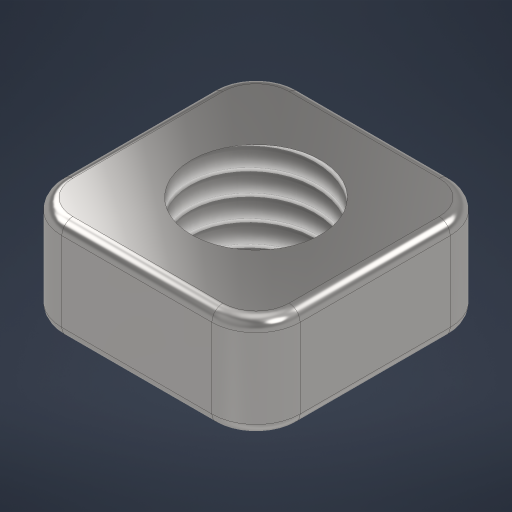
# Autodesk Inventor part: M3 Square Nut
Saved by Autodesk Inventor 2024 (Build 280153000, 153)
## iProperties
Created: 2024-10-26
Part Number: M3 Square Nut
Material: Generic
Document SubType Name: Modeling
Designer: jerem
Density: 1 g/cm^3
Appearance: Default
Author: jerem
Autodesk Inventor part; units mm, degrees
ref_plane "YZ Plane" through (0, 0, 0) normal (1, 0, 0) x (0, 1, 0)
ref_plane "XZ Plane" through (0, 0, 0) normal (0, 1, 0) x (-1, 0, 0)
ref_plane "XY Plane" through (0, 0, 0) normal (0, 0, 1) x (1, 0, 0)
sketch "Sketch1" plane through (0, 0, 0) normal (0, 1, 0) x (-1, 0, 0)
  circle A0 centre (0, 0) radius 1.465
  line L0 (-1.7, -2.7) -> (1.7, -2.7)
  line L1 (2.7, -1.7) -> (2.7, 1.7)
  line L2 (1.7, 2.7) -> (-1.7, 2.7)
  line L3 (-2.7, 1.7) -> (-2.7, -1.7)
  line L4 (-2.7, -2.7) -> (2.7, 2.7) construction
  line L5 (2.7, -2.7) -> (-2.7, 2.7) construction
  arc A1 (2.7, 1.7) -> (1.7, 2.7) centre (1.7, 1.7) ccw
  arc A2 (-1.7, 2.7) -> (-2.7, 1.7) centre (-1.7, 1.7) ccw
  arc A3 (-2.7, -1.7) -> (-1.7, -2.7) centre (-1.7, -1.7) ccw
  arc A4 (1.7, -2.7) -> (2.7, -1.7) centre (1.7, -1.7) ccw
  dimension "d0" = 2.93
  dimension "d1" = 5.4
  dimension "d2" = 5.4
  dimension "d3" = 1
  constraints: 12 end point, 8 point on circle, 8 point on line, 8 tangent, 5 centre point, 3 equal radius, 2 midpoint, 2 parallel, 1 coincident, 1 horizontal, 1 perpendicular
  measures "d0" diameter of A0
  measures "d1" distance of L5.end L4.end
  measures "d2" distance of L4.end L5.start
  measures "d3" radius of A1
extrude "Extrusion1" add sketch "Sketch1" along normal blind 2.3
fillet "Fillet1" radius 0.25 16 edges at (2.7, 2.3, 0) (2.4071, 2.3, -2.4071) (0, 2.3, -2.7) (-2.4071, 2.3, -2.4071) (-2.7, 2.3, 0) (-2.4071, 2.3, 2.4071) (0, 2.3, 2.7) (2.4071, 2.3, 2.4071) (2.7, 0, 0) (2.4071, 0, -2.4071) (0, 0, -2.7) (-2.4071, 0, -2.4071) (-2.7, 0, 0) (-2.4071, 0, 2.4071) (0, 0, 2.7) (2.4071, 0, 2.4071)
thread "Thread1" size "M3x0.5" class "6H" standard "ANSI Metric M Profile" full length
body "Solid1"
